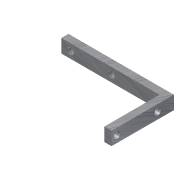
# Autodesk Inventor part: Pelvis
Saved by Autodesk Inventor 2011 (Build 150239000, 239)
## iProperties
Created: 2010-11-21
Part Number: Pelvis
Document SubType Name: Modeling
Designer: Milton
Density: 2.71 g/cm^3
Mass: 2.86426 g
Surface Area: 12.4201 cm^2
Volume: 1.05692 cm^3
Material: Aluminum-6061
Author: Milton
Autodesk Inventor part; units mm, degrees
ref_plane "YZ Plane" through (0, 0, 0) normal (1, 0, 0) x (0, 1, 0)
ref_plane "XZ Plane" through (0, 0, 0) normal (0, 1, 0) x (-1, 0, 0)
ref_plane "XY Plane" through (0, 0, 0) normal (0, 0, 1) x (1, 0, 0)
sketch "Sketch1" plane through (0, 0, 0) normal (0, 0, 1) x (1, 0, 0)
  line L0 (56.3662, 12.7852) -> (56.3662, 35.7852)
  line L1 (56.3662, 35.7852) -> (15.3628, 35.7852)
  line L2 (15.3628, 35.7852) -> (15.3662, 38.7852)
  line L3 (15.3662, 38.7852) -> (59.3662, 38.7852)
  line L4 (59.3662, 38.7852) -> (59.3662, 12.7852)
  line L5 (56.3662, 12.7852) -> (59.3662, 12.7852)
  point P0 (0, 0)
  dimension "d0" = 3
  dimension "d1" = 3
  dimension "d2" = 26
  dimension "d3" = 44
  constraints: 12 end point, 2 horizontal, 2 vertical, 1 perpendicular
  measures "d0" distance of L1.end L2.end
  measures "d1" distance of L0.start L4.end
  measures "d2" distance of L3.end L4.end
  measures "d3" distance of L2.end L3.end
extrude "Extrusion1" add sketch "Sketch1" along normal blind 5.6
sketch "Sketch2" plane through (56.3662, 12.7852, 0) normal (-1, 0, 0) x (0, 0, 1)
  circle A0 centre (2.8, 19.3) radius 1.35 projected
  circle A1 centre (2.8, 2.3) radius 1.35 projected
  circle A2 centre (2.8, 19.3) radius 1.35
  circle A3 centre (2.8, 2.3) radius 1.35
  point P0 (0, -12.7852)
  dimension "d6" = 2.7
  dimension "d7" = 2.7
  constraints: 2 centre point, 2 coincident
  measures "d6" diameter of A2
  measures "d7" diameter of A3
extrude "Extrusion2" cut sketch "Sketch2" against normal through all
sketch "Sketch3" plane through (15.3628, 35.7852, 0) normal (0, -1, 0) x (1, 0, 0)
  circle A0 centre (3.9023, 2.8) radius 1.35 projected
  circle A1 centre (20.9023, 2.8) radius 1.35 projected
  circle A2 centre (3.9023, 2.8) radius 1.35
  circle A3 centre (20.9023, 2.8) radius 1.35
  point P0 (-15.3628, 0)
  dimension "d10" = 2.7
  dimension "d11" = 2.7
  constraints: 2 centre point, 2 coincident, 1 concentric
  measures "d10" diameter of A3
  measures "d11" diameter of A2
extrude "Extrusion3" cut sketch "Sketch3" against normal through all
body "Solid1"
